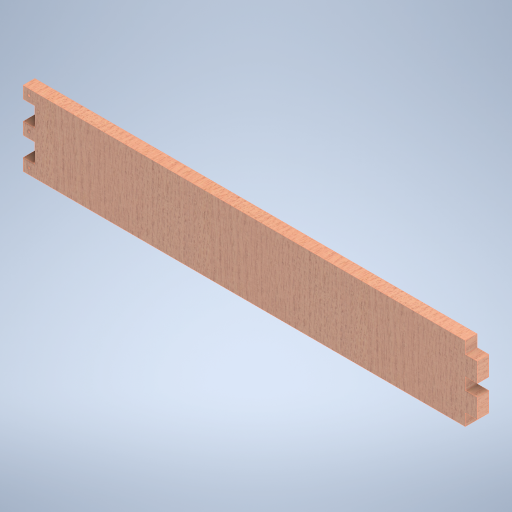
# Autodesk Inventor part: Bumper wood
Saved by Autodesk Inventor 2023 (Build 270158000, 158)
## iProperties
Created: 2023-11-22
Part Number: Bumper wood
Material: Wood (Oak)
Document SubType Name: Modeling
Designer: adamarnold
Density: 0.76 g/cm^3
Appearance: White Oak - Natural Medium Gloss
Author: adamarnold
Autodesk Inventor part; units mm, degrees
ref_plane "YZ Plane" through (0, 0, 0) normal (1, 0, 0) x (0, 1, 0)
ref_plane "XZ Plane" through (0, 0, 0) normal (0, 1, 0) x (-1, 0, 0)
ref_plane "XY Plane" through (0, 0, 0) normal (0, 0, 1) x (1, 0, 0)
sketch "Sketch1" plane through (0, 0, 0) normal (0, 0, 1) x (1, 0, 0)
  line L0 (0, 0) -> (-735.0125, 0)
  line L1 (-735.0125, 0) -> (-735.0125, 120.65)
  line L2 (-735.0125, 120.65) -> (0, 120.65)
  line L3 (0, 120.65) -> (0, 0)
  dimension "d0" = 735.0125
  dimension "d1" = 120.65
  constraints: 8 end point, 2 parallel, 1 horizontal, 1 perpendicular
  measures "d0" distance of L1.end L2.end
  measures "d1" distance of L0.end L1.end
extrude "Extrusion1" add sketch "Sketch1" along normal blind 19.05
sketch "Sketch2" plane through (0, 0, 19.05) normal (0, 0, 1) x (1, 0, 0)
  line L0 (0, 120.65) -> (-735.0125, 120.65) projected
  line L1 (0, 120.65) -> (-19.304, 120.65)
  line L2 (-19.304, 120.65) -> (-19.304, 101.346)
  line L3 (-19.304, 101.346) -> (0, 101.346)
  line L4 (0, 101.346) -> (0, 120.65)
  line L5 (0, 0) -> (-19.304, 0)
  line L6 (-19.304, 0) -> (-19.304, 19.304)
  line L7 (-19.304, 19.304) -> (0, 19.304)
  line L8 (0, 19.304) -> (0, 0)
  line L9 (0, 0) -> (0, 120.65) projected
  line L10 (0, 60.325) -> (-19.304, 60.325)
  line L11 (0, 69.977) -> (-19.304, 69.977)
  line L12 (0, 50.673) -> (-19.304, 50.673)
  line L13 (-19.304, 69.977) -> (-19.304, 50.673)
  line L14 (0, 69.977) -> (0, 50.673)
  line L15 (-735.0125, 120.65) -> (-735.0125, 0) projected
  line L16 (-735.0125, 120.65) -> (-735.0125, 101.346)
  line L17 (-735.0125, 101.346) -> (-715.7085, 101.346)
  line L18 (-715.7085, 101.346) -> (-735.0125, 101.346)
  line L19 (-735.0125, 101.346) -> (-735.0125, 69.977)
  line L20 (-735.0125, 69.977) -> (-715.7085, 69.977)
  line L21 (-715.7085, 69.977) -> (-715.7085, 101.346)
  line L22 (-735.0125, 60.325) -> (-720.7714, 60.325)
  line L23 (-735.0125, 0) -> (-735.0125, 120.65)
  line L24 (-735.0125, 0) -> (-735.0125, 19.304)
  line L25 (-735.0125, 19.304) -> (-715.7085, 19.304)
  line L26 (-715.7085, 19.304) -> (-735.0125, 19.304)
  line L27 (-735.0125, 19.304) -> (-735.0125, 50.673)
  line L28 (-735.0125, 50.673) -> (-715.7085, 50.673)
  line L29 (-715.7085, 50.673) -> (-715.7085, 19.304)
  circle A0 centre (-725.3605, 110.998) radius 1.5875
  circle A1 centre (-725.3605, 60.325) radius 1.5875
  circle A2 centre (-725.3605, 9.652) radius 1.5875
  line L30 (-735.0125, 0) -> (0, 0) projected
  point P0 (-735.0125, 19.304)
  point P1 (-725.3605, 101.346)
  point P2 (-725.3605, 101.346)
  dimension "d4" = 19.304
  dimension "d5" = 19.304
  dimension "d6" = 19.304
  dimension "d7" = 19.304
  dimension "d8" = 19.304
  dimension "d9" = 9.652
  dimension "d10" = 9.652
  dimension "d14" = 19.304
  dimension "d15" = 19.304
  dimension "d16" = 31.369
  dimension "d31" = 9.652
  dimension "d32" = 9.652
  dimension "d33" = 3.175
  constraints: 54 end point, 9 parallel, 7 symmetric about line, 5 horizontal, 5 midpoint, 5 point on line, 4 perpendicular, 3 centre point, 3 vertical alignment, 2 equal radius, 1 horizontal alignment, 1 vertical
  measures "d4" distance of L3.end L2.end
  measures "d5" distance of L2.end L1.end
  measures "d6" distance of L6.end L7.end
  measures "d7" distance of L5.end L6.end
  measures "d8" distance of L10.start L10.end
  measures "d9" distance between parallel lines of L10 L11
  measures "d10" distance between parallel lines of L10 L12
  measures "d14" distance of L0.end L16.end
  measures "d15" distance of L16.end L17.end
  measures "d16" distance of L19.end L18.end
  measures "d31" distance from line of L0 A0.centre
  measures "d32" distance from line of A2.centre L30
  measures "d33" diameter of A0
extrude "Extrusion2" cut sketch "Sketch2" against normal through all contours L4 L3 L2 L0 | A1 L22 | L22 A1 | L9 L10 L13 L11 | L17 L21 L20 L15 | L9 L12 L13 L10 | L8 L5 L6 L7 | L28 L29 L25 L15 | A0 | A2
sketch "Sketch3" plane through (0, 0, 19.05) normal (0, 0, 1) x (1, 0, 0)
  line L0 (-735.0125, 120.65) -> (-735.0125, 101.346) projected
  line L1 (-368.3, 120.65) -> (-368.3, 18.5529)
  line L2 (-368.3, 95.25) -> (-287.1671, 95.25)
  line L3 (-368.3, 76.2) -> (-321.3262, 76.2)
  line L4 (-368.3, 57.15) -> (-321.3262, 57.15)
  line L5 (-715.7085, 101.346) -> (-715.7085, 69.977) projected
  line L6 (-715.7085, 101.346) -> (-715.7085, 120.65)
  point P0 (0, 0)
  point P1 (-327.7336, 95.25)
  point P2 (-715.7085, 110.998)
  dimension "d30" = 347.4085
  constraints: 10 end point, 3 horizontal, 3 point on line, 2 midpoint, 1 vertical
  measures "d30" distance from line of L1 point (-715.708, 110.998)
hole "Hole1" [suppressed]
equation "\"d31\" = 0.5 * d14"
equation "\"d32\" = d31"
body "Solid1"
